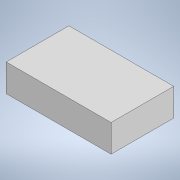
# Autodesk Inventor part: Battery
Saved by Autodesk Inventor 2020 (Build 240168000, 168)
## iProperties
Created: 2021-11-16
Part Number: Battery
Material: Generic
Document SubType Name: Modeling
Designer: mtkts
Density: 1 g/cm^3
Appearance: Default
Author: mtkts
Autodesk Inventor part; units mm, degrees
ref_plane "YZ Plane" through (0, 0, 0) normal (1, 0, 0) x (0, 1, 0)
ref_plane "XZ Plane" through (0, 0, 0) normal (0, 1, 0) x (-1, 0, 0)
ref_plane "XY Plane" through (0, 0, 0) normal (0, 0, 1) x (1, 0, 0)
sketch "Sketch1" plane through (0, 0, 0) normal (0, 1, 0) x (-1, 0, 0)
  line L0 (-20.828, 12.446) -> (20.828, 12.446)
  line L1 (20.828, 12.446) -> (20.828, -12.446)
  line L2 (20.828, -12.446) -> (-20.828, -12.446)
  line L3 (-20.828, -12.446) -> (-20.828, 12.446)
  line L4 (-20.828, 12.446) -> (20.828, -12.446) construction
  line L5 (20.828, 12.446) -> (-20.828, -12.446) construction
  point P0 (0, 0)
  dimension "d0" = 41.656
  dimension "d1" = 24.892
  constraints: 12 end point, 2 midpoint, 2 parallel, 1 horizontal, 1 perpendicular
  measures "d0" distance of L1.end L2.end
  measures "d1" distance of L0.end L1.end
extrude "Extrusion1" add sketch "Sketch1" along normal blind 10.922
body "Solid1"
